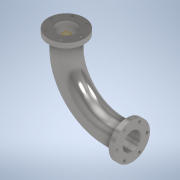
# Autodesk Inventor part: Parametric
Saved by Autodesk Inventor 2022 (Build 260153000, 153)
## iProperties
Created: 2022-02-07
Part Number: Parametric
Material: Steel, Mild
Document SubType Name: Modeling
Designer: joshw
Density: 7.85 g/cm^3
Appearance: Semi-Polished
Author: joshw
Autodesk Inventor part; units mm, degrees
ref_plane "YZ Plane" through (0, 0, 0) normal (1, 0, 0) x (0, 1, 0)
ref_plane "XZ Plane" through (0, 0, 0) normal (0, 1, 0) x (-1, 0, 0)
ref_plane "XY Plane" through (0, 0, 0) normal (0, 0, 1) x (1, 0, 0)
sketch "Sketch1" plane through (0, 0, 0) normal (0, 0, 1) x (1, 0, 0)
  line L0 (-265.2211, 0) -> (0, 0)
  line L1 (0, 0) -> (0, -436.8243)
  arc A0 (-200, 0) -> (0, -200) centre (0, 0) ccw
  line L2 (-200, 0) -> (-200, 50)
  line L3 (0, -200) -> (50, -200)
  dimension "d30" = 400
  dimension "d31" = 50
  dimension "d32" = 50
  constraints: 8 end point, 3 perpendicular, 2 coincident, 2 point on circle, 2 point on line, 2 tangent, 1 centre point, 1 horizontal
  measures "d30" diameter of A0
  measures "d31" distance of L2.start L2.end
  measures "d32" distance of L3.start L3.end
ref_plane "Work Plane1" through (-200, 50, 0) normal (0, 1, 0) x (-1, 0, 0)
sketch "Sketch2" plane through (-200, 50, 0) normal (0, 1, 0) x (-1, 0, 0)
  circle A0 centre (0, 0) radius 75
  circle A1 centre (0, 0) radius 37.5
  circle A2 centre (62.5, 0) radius 5
  circle A3 centre (31.25, 54.1266) radius 5
  circle A4 centre (-31.25, 54.1266) radius 5
  circle A5 centre (-62.5, 0) radius 5
  circle A6 centre (-31.25, -54.1266) radius 5
  circle A7 centre (31.25, -54.1266) radius 5
  point P0 (-200, 0)
  dimension "d3" = 150
  dimension "d4" = 75
  dimension "d5" = 10
  dimension "d6" = 62.5
  dimension "d9" = 360
  constraints: 8 centre point, 1 coincident, 13 other
  measures "d3" diameter of A0
  measures "d4" diameter of A1
  measures "d5" diameter of A2
  measures "d6" distance of A0.centre A2.centre
sketch "Sketch3" plane through (-200, 50, 0) normal (0, 1, 0) x (-1, 0, 0)
  circle A0 centre (0, 0) radius 50
  circle A1 centre (0, 0) radius 37.5
  point P0 (-200, 0)
  dimension "d11" = 100
  dimension "d12" = 75
  constraints: 2 centre point, 1 coincident
  measures "d11" diameter of A0
  measures "d12" diameter of A1
sweep "Sweep2" add profiles "Sketch3" path "Sketch1" path curves L2 A0 L3
extrude "Extrusion3" add sketch "Sketch2" along normal blind 20
sketch "Sketch5" plane through (50, -200, 0) normal (1, 0, 0) x (0, 0, -1)
  circle A0 centre (0, 0) radius 75
  circle A1 centre (0, 0) radius 37.5
  circle A2 centre (62.5, 0) radius 5
  circle A3 centre (31.25, 54.1266) radius 5
  circle A4 centre (-31.25, 54.1266) radius 5
  circle A5 centre (-62.5, 0) radius 5
  circle A6 centre (-31.25, -54.1266) radius 5
  circle A7 centre (31.25, -54.1266) radius 5
  point P0 (0, 200)
  dimension "d39" = 150
  dimension "d40" = 75
  dimension "d41" = 10
  dimension "d42" = 62.5
  dimension "d43" = 360
  constraints: 8 centre point, 1 coincident, 13 other
  measures "d39" diameter of A0
  measures "d40" diameter of A1
  measures "d41" diameter of A2
  measures "d42" distance of A0.centre A2.centre
extrude "Extrusion4" add sketch "Sketch5" along normal blind 20
equation "\"d30\" = Elbow_Diameter"
equation "\"d31\" = Elbow_Length"
equation "\"d32\" = Elbow_Length"
equation "\"d3\" = Flange_Diameter"
equation "\"d4\" = Inner_Diameter"
equation "\"d5\" = Hole_Diameter"
equation "\"d6\" = Hole_Position"
equation "\"d11\" = Outer_Diameter"
equation "\"d12\" = Inner_Diameter"
equation "\"d35\" = Flange_Hight"
equation "\"d39\" = Flange_Diameter"
equation "\"d40\" = Inner_Diameter"
equation "\"d41\" = Hole_Diameter"
equation "\"d42\" = Hole_Position"
equation "\"d48\" = Flange_Hight"
equation "\"Elbow_Diameter\" = 400"
equation "\"Elbow_Length\" = 50"
equation "\"Flange_Diameter\" = 150"
equation "\"Inner_Diameter\" = 75"
equation "\"Fillet_Radius\" = 6"
equation "\"Flange_Hight\" = 20"
equation "\"Hole_Position\" = 0.166667 * Inner_Diameter + 0.333333 * Flange_Diameter"
equation "\"Hole_Diameter\" = 10"
equation "\"Outer_Diameter\" = 100"
body "Solid2"
